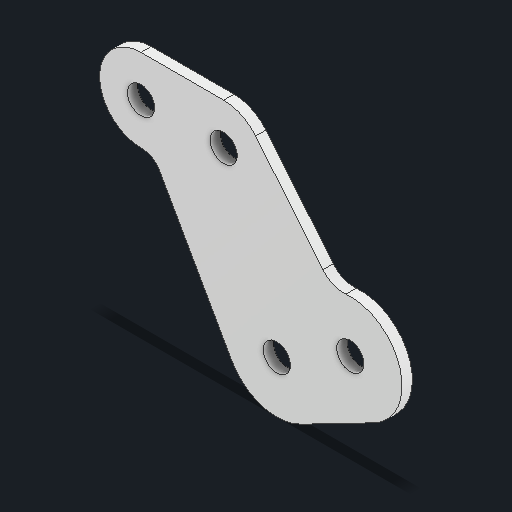
# Autodesk Inventor part: Clamp Gusset
Saved by Autodesk Inventor 2025.1 (Build 291241000, 241)
## iProperties
Created: 2024-11-12
Part Number: Clamp Gusset
Material: Acetal Resin, White
Document SubType Name: Modeling
Designer: avere
Density: 1.425 g/cm^3
Appearance: Smooth - White
Author: avere
Autodesk Inventor part; units mm, degrees
ref_plane "YZ Plane" through (0, 0, 0) normal (1, 0, 0) x (0, 1, 0)
ref_plane "XZ Plane" through (0, 0, 0) normal (0, 1, 0) x (-1, 0, 0)
ref_plane "XY Plane" through (0, 0, 0) normal (0, 0, 1) x (1, 0, 0)
sketch "Sketch1" plane through (0, 0, 0) normal (0, 0, 1) x (1, 0, 0)
  circle A0 centre (0, 0) radius 2.0955
  circle A1 centre (-12.7, 0) radius 2.0955
  arc A2 (-12.7, 6.35) -> (-12.7, -6.35) centre (-12.7, 0) ccw
  arc A3 (4.9096, 4.0272) -> (0, 6.35) centre (0, 0) ccw
  line L0 (0, 0) -> (32.8335, 0) construction
  line L1 (-12.6049, -6.35) -> (-12.7, -6.35)
  line L2 (-12.7, 6.35) -> (0, 6.35)
  line L3 (1.2503, -27.6905) -> (-9.8373, -7.969)
  arc A4 (-9.8373, -7.969) -> (-12.6049, -6.35) centre (-12.6049, -9.525) ccw
  arc A5 (1.2503, -27.6905) -> (11.8106, -30.8536) centre (8.1692, -23.8006) ccw
  circle A6 centre (8.1692, -23.8006) radius 2.0955
  circle A7 centre (19.454, -17.9745) radius 2.0955
  arc A8 (23.0953, -25.0275) -> (18.7723, -10.0663) centre (19.454, -17.9745) ccw
  line L4 (11.8106, -30.8536) -> (23.0953, -25.0275)
  arc A9 (15.2536, -8.5832) -> (18.7723, -10.0663) centre (18.4204, -5.9855) ccw
  line L5 (15.2536, -8.5832) -> (4.9096, 4.0272)
  point P0 (-10.4687, -6.35)
  dimension "d0" = 4.191
  dimension "d9" = 3.175
  dimension "d10" = 7.9375
  dimension "d11" = 4.191
  dimension "d13" = 4.191
  dimension "d14" = 15.875
  dimension "d15" = 12.7
  constraints: 12 end point, 12 point on circle, 10 centre point, 8 tangent, 5 coincident, 2 horizontal, 1 point on line, 3 other
  measures "d0" diameter of A0
  measures "d9" radius of A4
  measures "d10" radius of A5
  measures "d11" diameter of A6
  measures "d13" diameter of A7
  measures "d14" diameter of A8
  measures "d15" distance of A6.centre A8.centre
extrude "Extrusion1" add sketch "Sketch1" along normal blind 1.5875
body "Solid1"
